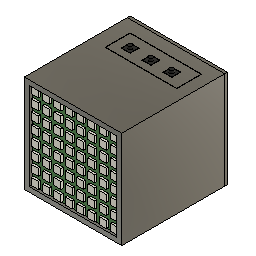
Enclosure (Autodesk Fusion 360 design; units mm, degrees)
Autodesk Fusion 360 part; units mm, degrees
sketch "Sketch1" plane through (0, 0, 0) normal (0, 1, 0) x (1, 0, 0) in component "LED Matrix"
  line L0 (32.5, 32.5) -> (-32.5, 32.5)
  line L1 (-32.5, 32.5) -> (-32.5, -32.5)
  line L2 (-32.5, -32.5) -> (32.5, -32.5)
  line L3 (32.5, -32.5) -> (32.5, 32.5)
  line L4 (32.5, 32.5) -> (-32.5, -32.5) construction
  line L5 (-32.5, 32.5) -> (32.5, -32.5) construction
  line L6 (31, 31) -> (-31, 31)
  line L7 (-31, 31) -> (-31, -31)
  line L8 (-31, -31) -> (31, -31)
  line L9 (31, -31) -> (31, 31)
  dimension "d1" = 65
  dimension "d2" = 65
  constraint parallel L0 L6
  constraint parallel L1 L7
  constraint parallel L2 L8
  constraint parallel L3 L9
  measures "d1" distance of L1.end L2.end
  measures "d2" distance of L0.end L1.end
extrude "Extrude1" add sketch "Sketch1" along normal blind 1.5 contours L0 L1 L2 L3 | L6 L7 L8 L9 makes body 1 in component "LED Matrix"
sketch "Sketch2" plane through (0, 0, 0) normal (0, -1, 0) x (1, 0, 0) in component "LED Matrix"
  line L0 (32.5, -32.5) -> (32.5, 32.5)
  line L1 (32.5, 32.5) -> (-32.5, 32.5)
  line L2 (-32.5, 32.5) -> (-32.5, -32.5)
  line L3 (-32.5, -32.5) -> (32.5, -32.5)
  line L4 (-31, -31) -> (-31, 31)
  line L5 (-31, 31) -> (31, 31)
  line L6 (31, 31) -> (31, -31)
  line L7 (31, -31) -> (-31, -31)
  line L8 (-31, 31) -> (-26, 31)
  line L9 (-26, 31) -> (-26, 26)
  line L10 (-26, 26) -> (-31, 26)
  line L11 (-31, 26) -> (-31, 31)
  line L12 (-22.8571, 31) -> (-17.8571, 31)
  line L13 (-22.8571, 26) -> (-22.8571, 31)
  line L14 (-17.8571, 26) -> (-22.8571, 26)
  line L15 (-17.8571, 31) -> (-17.8571, 26)
  line L16 (-14.7143, 31) -> (-9.7143, 31)
  line L17 (-14.7143, 26) -> (-14.7143, 31)
  line L18 (-9.7143, 26) -> (-14.7143, 26)
  line L19 (-9.7143, 31) -> (-9.7143, 26)
  line L20 (-6.5714, 31) -> (-1.5714, 31)
  line L21 (-6.5714, 26) -> (-6.5714, 31)
  line L22 (-1.5714, 26) -> (-6.5714, 26)
  line L23 (-1.5714, 31) -> (-1.5714, 26)
  line L24 (1.5714, 31) -> (6.5714, 31)
  line L25 (1.5714, 26) -> (1.5714, 31)
  line L26 (6.5714, 26) -> (1.5714, 26)
  line L27 (6.5714, 31) -> (6.5714, 26)
  line L28 (9.7143, 31) -> (14.7143, 31)
  line L29 (9.7143, 26) -> (9.7143, 31)
  line L30 (14.7143, 26) -> (9.7143, 26)
  line L31 (14.7143, 31) -> (14.7143, 26)
  line L32 (17.8571, 31) -> (22.8571, 31)
  line L33 (17.8571, 26) -> (17.8571, 31)
  line L34 (22.8571, 26) -> (17.8571, 26)
  line L35 (22.8571, 31) -> (22.8571, 26)
  line L36 (26, 31) -> (31, 31)
  line L37 (26, 26) -> (26, 31)
  line L38 (31, 26) -> (26, 26)
  line L39 (31, 31) -> (31, 26)
  line L40 (-31, 22.8571) -> (-26, 22.8571)
  line L41 (-31, 17.8571) -> (-31, 22.8571)
  line L42 (-26, 17.8571) -> (-31, 17.8571)
  line L43 (-26, 22.8571) -> (-26, 17.8571)
  line L44 (-22.8571, 22.8571) -> (-17.8571, 22.8571)
  line L45 (-22.8571, 17.8571) -> (-22.8571, 22.8571)
  line L46 (-17.8571, 17.8571) -> (-22.8571, 17.8571)
  line L47 (-17.8571, 22.8571) -> (-17.8571, 17.8571)
  line L48 (-14.7143, 22.8571) -> (-9.7143, 22.8571)
  line L49 (-14.7143, 17.8571) -> (-14.7143, 22.8571)
  line L50 (-9.7143, 17.8571) -> (-14.7143, 17.8571)
  line L51 (-9.7143, 22.8571) -> (-9.7143, 17.8571)
  line L52 (-6.5714, 22.8571) -> (-1.5714, 22.8571)
  line L53 (-6.5714, 17.8571) -> (-6.5714, 22.8571)
  line L54 (-1.5714, 17.8571) -> (-6.5714, 17.8571)
  line L55 (-1.5714, 22.8571) -> (-1.5714, 17.8571)
  line L56 (1.5714, 22.8571) -> (6.5714, 22.8571)
  line L57 (1.5714, 17.8571) -> (1.5714, 22.8571)
  line L58 (6.5714, 17.8571) -> (1.5714, 17.8571)
  line L59 (6.5714, 22.8571) -> (6.5714, 17.8571)
  line L60 (9.7143, 22.8571) -> (14.7143, 22.8571)
  line L61 (9.7143, 17.8571) -> (9.7143, 22.8571)
  line L62 (14.7143, 17.8571) -> (9.7143, 17.8571)
  line L63 (14.7143, 22.8571) -> (14.7143, 17.8571)
  line L64 (17.8571, 22.8571) -> (22.8571, 22.8571)
  line L65 (17.8571, 17.8571) -> (17.8571, 22.8571)
  line L66 (22.8571, 17.8571) -> (17.8571, 17.8571)
  line L67 (22.8571, 22.8571) -> (22.8571, 17.8571)
  line L68 (26, 22.8571) -> (31, 22.8571)
  line L69 (26, 17.8571) -> (26, 22.8571)
  line L70 (31, 17.8571) -> (26, 17.8571)
  line L71 (31, 22.8571) -> (31, 17.8571)
  line L72 (-31, 14.7143) -> (-26, 14.7143)
  line L73 (-31, 9.7143) -> (-31, 14.7143)
  line L74 (-26, 9.7143) -> (-31, 9.7143)
  line L75 (-26, 14.7143) -> (-26, 9.7143)
  line L76 (-22.8571, 14.7143) -> (-17.8571, 14.7143)
  line L77 (-22.8571, 9.7143) -> (-22.8571, 14.7143)
  line L78 (-17.8571, 9.7143) -> (-22.8571, 9.7143)
  line L79 (-17.8571, 14.7143) -> (-17.8571, 9.7143)
  line L80 (-14.7143, 14.7143) -> (-9.7143, 14.7143)
  line L81 (-14.7143, 9.7143) -> (-14.7143, 14.7143)
  line L82 (-9.7143, 9.7143) -> (-14.7143, 9.7143)
  line L83 (-9.7143, 14.7143) -> (-9.7143, 9.7143)
  line L84 (-6.5714, 14.7143) -> (-1.5714, 14.7143)
  line L85 (-6.5714, 9.7143) -> (-6.5714, 14.7143)
  line L86 (-1.5714, 9.7143) -> (-6.5714, 9.7143)
  line L87 (-1.5714, 14.7143) -> (-1.5714, 9.7143)
  line L88 (1.5714, 14.7143) -> (6.5714, 14.7143)
  line L89 (1.5714, 9.7143) -> (1.5714, 14.7143)
  line L90 (6.5714, 9.7143) -> (1.5714, 9.7143)
  line L91 (6.5714, 14.7143) -> (6.5714, 9.7143)
  line L92 (9.7143, 14.7143) -> (14.7143, 14.7143)
  line L93 (9.7143, 9.7143) -> (9.7143, 14.7143)
  line L94 (14.7143, 9.7143) -> (9.7143, 9.7143)
  line L95 (14.7143, 14.7143) -> (14.7143, 9.7143)
  line L96 (17.8571, 14.7143) -> (22.8571, 14.7143)
  line L97 (17.8571, 9.7143) -> (17.8571, 14.7143)
  line L98 (22.8571, 9.7143) -> (17.8571, 9.7143)
  line L99 (22.8571, 14.7143) -> (22.8571, 9.7143)
  line L100 (26, 14.7143) -> (31, 14.7143)
  line L101 (26, 9.7143) -> (26, 14.7143)
  line L102 (31, 9.7143) -> (26, 9.7143)
  line L103 (31, 14.7143) -> (31, 9.7143)
  line L104 (-31, 6.5714) -> (-26, 6.5714)
  line L105 (-31, 1.5714) -> (-31, 6.5714)
  line L106 (-26, 1.5714) -> (-31, 1.5714)
  line L107 (-26, 6.5714) -> (-26, 1.5714)
  line L108 (-22.8571, 6.5714) -> (-17.8571, 6.5714)
  line L109 (-22.8571, 1.5714) -> (-22.8571, 6.5714)
  line L110 (-17.8571, 1.5714) -> (-22.8571, 1.5714)
  line L111 (-17.8571, 6.5714) -> (-17.8571, 1.5714)
  line L112 (-14.7143, 6.5714) -> (-9.7143, 6.5714)
  line L113 (-14.7143, 1.5714) -> (-14.7143, 6.5714)
  line L114 (-9.7143, 1.5714) -> (-14.7143, 1.5714)
  line L115 (-9.7143, 6.5714) -> (-9.7143, 1.5714)
  line L116 (-6.5714, 6.5714) -> (-1.5714, 6.5714)
  line L117 (-6.5714, 1.5714) -> (-6.5714, 6.5714)
  line L118 (-1.5714, 1.5714) -> (-6.5714, 1.5714)
  line L119 (-1.5714, 6.5714) -> (-1.5714, 1.5714)
  line L120 (1.5714, 6.5714) -> (6.5714, 6.5714)
  line L121 (1.5714, 1.5714) -> (1.5714, 6.5714)
  line L122 (6.5714, 1.5714) -> (1.5714, 1.5714)
  line L123 (6.5714, 6.5714) -> (6.5714, 1.5714)
  line L124 (9.7143, 6.5714) -> (14.7143, 6.5714)
  line L125 (9.7143, 1.5714) -> (9.7143, 6.5714)
  line L126 (14.7143, 1.5714) -> (9.7143, 1.5714)
  line L127 (14.7143, 6.5714) -> (14.7143, 1.5714)
  line L128 (17.8571, 6.5714) -> (22.8571, 6.5714)
  line L129 (17.8571, 1.5714) -> (17.8571, 6.5714)
  line L130 (22.8571, 1.5714) -> (17.8571, 1.5714)
  line L131 (22.8571, 6.5714) -> (22.8571, 1.5714)
  line L132 (26, 6.5714) -> (31, 6.5714)
  line L133 (26, 1.5714) -> (26, 6.5714)
  line L134 (31, 1.5714) -> (26, 1.5714)
  line L135 (31, 6.5714) -> (31, 1.5714)
  line L136 (-31, -1.5714) -> (-26, -1.5714)
  line L137 (-31, -6.5714) -> (-31, -1.5714)
  line L138 (-26, -6.5714) -> (-31, -6.5714)
  line L139 (-26, -1.5714) -> (-26, -6.5714)
  line L140 (-22.8571, -1.5714) -> (-17.8571, -1.5714)
  line L141 (-22.8571, -6.5714) -> (-22.8571, -1.5714)
  line L142 (-17.8571, -6.5714) -> (-22.8571, -6.5714)
  line L143 (-17.8571, -1.5714) -> (-17.8571, -6.5714)
  line L144 (-14.7143, -1.5714) -> (-9.7143, -1.5714)
  line L145 (-14.7143, -6.5714) -> (-14.7143, -1.5714)
  line L146 (-9.7143, -6.5714) -> (-14.7143, -6.5714)
  line L147 (-9.7143, -1.5714) -> (-9.7143, -6.5714)
  line L148 (-6.5714, -1.5714) -> (-1.5714, -1.5714)
  line L149 (-6.5714, -6.5714) -> (-6.5714, -1.5714)
  line L150 (-1.5714, -6.5714) -> (-6.5714, -6.5714)
  line L151 (-1.5714, -1.5714) -> (-1.5714, -6.5714)
  line L152 (1.5714, -1.5714) -> (6.5714, -1.5714)
  line L153 (1.5714, -6.5714) -> (1.5714, -1.5714)
  line L154 (6.5714, -6.5714) -> (1.5714, -6.5714)
  line L155 (6.5714, -1.5714) -> (6.5714, -6.5714)
  line L156 (9.7143, -1.5714) -> (14.7143, -1.5714)
  line L157 (9.7143, -6.5714) -> (9.7143, -1.5714)
  line L158 (14.7143, -6.5714) -> (9.7143, -6.5714)
  line L159 (14.7143, -1.5714) -> (14.7143, -6.5714)
  line L160 (17.8571, -1.5714) -> (22.8571, -1.5714)
  line L161 (17.8571, -6.5714) -> (17.8571, -1.5714)
  line L162 (22.8571, -6.5714) -> (17.8571, -6.5714)
  line L163 (22.8571, -1.5714) -> (22.8571, -6.5714)
  line L164 (26, -1.5714) -> (31, -1.5714)
  line L165 (26, -6.5714) -> (26, -1.5714)
  line L166 (31, -6.5714) -> (26, -6.5714)
  line L167 (31, -1.5714) -> (31, -6.5714)
  line L168 (-31, -9.7143) -> (-26, -9.7143)
  line L169 (-31, -14.7143) -> (-31, -9.7143)
  line L170 (-26, -14.7143) -> (-31, -14.7143)
  line L171 (-26, -9.7143) -> (-26, -14.7143)
  line L172 (-22.8571, -9.7143) -> (-17.8571, -9.7143)
  line L173 (-22.8571, -14.7143) -> (-22.8571, -9.7143)
  line L174 (-17.8571, -14.7143) -> (-22.8571, -14.7143)
  line L175 (-17.8571, -9.7143) -> (-17.8571, -14.7143)
  line L176 (-14.7143, -9.7143) -> (-9.7143, -9.7143)
  line L177 (-14.7143, -14.7143) -> (-14.7143, -9.7143)
  line L178 (-9.7143, -14.7143) -> (-14.7143, -14.7143)
  line L179 (-9.7143, -9.7143) -> (-9.7143, -14.7143)
  line L180 (-6.5714, -9.7143) -> (-1.5714, -9.7143)
  line L181 (-6.5714, -14.7143) -> (-6.5714, -9.7143)
  line L182 (-1.5714, -14.7143) -> (-6.5714, -14.7143)
  line L183 (-1.5714, -9.7143) -> (-1.5714, -14.7143)
  line L184 (1.5714, -9.7143) -> (6.5714, -9.7143)
  line L185 (1.5714, -14.7143) -> (1.5714, -9.7143)
  line L186 (6.5714, -14.7143) -> (1.5714, -14.7143)
  line L187 (6.5714, -9.7143) -> (6.5714, -14.7143)
  line L188 (9.7143, -9.7143) -> (14.7143, -9.7143)
  line L189 (9.7143, -14.7143) -> (9.7143, -9.7143)
  line L190 (14.7143, -14.7143) -> (9.7143, -14.7143)
  line L191 (14.7143, -9.7143) -> (14.7143, -14.7143)
  line L192 (17.8571, -9.7143) -> (22.8571, -9.7143)
  line L193 (17.8571, -14.7143) -> (17.8571, -9.7143)
  line L194 (22.8571, -14.7143) -> (17.8571, -14.7143)
  line L195 (22.8571, -9.7143) -> (22.8571, -14.7143)
  line L196 (26, -9.7143) -> (31, -9.7143)
  line L197 (26, -14.7143) -> (26, -9.7143)
  line L198 (31, -14.7143) -> (26, -14.7143)
  line L199 (31, -9.7143) -> (31, -14.7143)
  line L200 (-31, -17.8571) -> (-26, -17.8571)
  line L201 (-31, -22.8571) -> (-31, -17.8571)
  line L202 (-26, -22.8571) -> (-31, -22.8571)
  line L203 (-26, -17.8571) -> (-26, -22.8571)
  line L204 (-22.8571, -17.8571) -> (-17.8571, -17.8571)
  line L205 (-22.8571, -22.8571) -> (-22.8571, -17.8571)
  line L206 (-17.8571, -22.8571) -> (-22.8571, -22.8571)
  line L207 (-17.8571, -17.8571) -> (-17.8571, -22.8571)
  line L208 (-14.7143, -17.8571) -> (-9.7143, -17.8571)
  line L209 (-14.7143, -22.8571) -> (-14.7143, -17.8571)
  line L210 (-9.7143, -22.8571) -> (-14.7143, -22.8571)
  line L211 (-9.7143, -17.8571) -> (-9.7143, -22.8571)
  line L212 (-6.5714, -17.8571) -> (-1.5714, -17.8571)
  line L213 (-6.5714, -22.8571) -> (-6.5714, -17.8571)
  line L214 (-1.5714, -22.8571) -> (-6.5714, -22.8571)
  line L215 (-1.5714, -17.8571) -> (-1.5714, -22.8571)
  line L216 (1.5714, -17.8571) -> (6.5714, -17.8571)
  line L217 (1.5714, -22.8571) -> (1.5714, -17.8571)
  line L218 (6.5714, -22.8571) -> (1.5714, -22.8571)
  line L219 (6.5714, -17.8571) -> (6.5714, -22.8571)
  line L220 (9.7143, -17.8571) -> (14.7143, -17.8571)
  line L221 (9.7143, -22.8571) -> (9.7143, -17.8571)
  line L222 (14.7143, -22.8571) -> (9.7143, -22.8571)
  line L223 (14.7143, -17.8571) -> (14.7143, -22.8571)
  line L224 (17.8571, -17.8571) -> (22.8571, -17.8571)
  line L225 (17.8571, -22.8571) -> (17.8571, -17.8571)
  line L226 (22.8571, -22.8571) -> (17.8571, -22.8571)
  line L227 (22.8571, -17.8571) -> (22.8571, -22.8571)
  line L228 (26, -17.8571) -> (31, -17.8571)
  line L229 (26, -22.8571) -> (26, -17.8571)
  line L230 (31, -22.8571) -> (26, -22.8571)
  line L231 (31, -17.8571) -> (31, -22.8571)
  line L232 (-31, -26) -> (-26, -26)
  line L233 (-31, -31) -> (-31, -26)
  line L234 (-26, -31) -> (-31, -31)
  line L235 (-26, -26) -> (-26, -31)
  line L236 (-22.8571, -26) -> (-17.8571, -26)
  line L237 (-22.8571, -31) -> (-22.8571, -26)
  line L238 (-17.8571, -31) -> (-22.8571, -31)
  line L239 (-17.8571, -26) -> (-17.8571, -31)
  line L240 (-14.7143, -26) -> (-9.7143, -26)
  line L241 (-14.7143, -31) -> (-14.7143, -26)
  line L242 (-9.7143, -31) -> (-14.7143, -31)
  line L243 (-9.7143, -26) -> (-9.7143, -31)
  line L244 (-6.5714, -26) -> (-1.5714, -26)
  line L245 (-6.5714, -31) -> (-6.5714, -26)
  line L246 (-1.5714, -31) -> (-6.5714, -31)
  line L247 (-1.5714, -26) -> (-1.5714, -31)
  line L248 (1.5714, -26) -> (6.5714, -26)
  line L249 (1.5714, -31) -> (1.5714, -26)
  line L250 (6.5714, -31) -> (1.5714, -31)
  line L251 (6.5714, -26) -> (6.5714, -31)
  line L252 (9.7143, -26) -> (14.7143, -26)
  line L253 (9.7143, -31) -> (9.7143, -26)
  line L254 (14.7143, -31) -> (9.7143, -31)
  line L255 (14.7143, -26) -> (14.7143, -31)
  line L256 (17.8571, -26) -> (22.8571, -26)
  line L257 (17.8571, -31) -> (17.8571, -26)
  line L258 (22.8571, -31) -> (17.8571, -31)
  line L259 (22.8571, -26) -> (22.8571, -31)
  line L260 (26, -26) -> (31, -26)
  line L261 (26, -31) -> (26, -26)
  line L262 (31, -31) -> (26, -31)
  line L263 (31, -26) -> (31, -31)
  dimension "d12" = 57
  dimension "d13" = -57
  constraint horizontal L8
  constraint vertical L9
  constraint horizontal L10
  constraint vertical L11
  constraint coincident L4.end L5.start
extrude "Extrude2" add sketch "Sketch2" along normal blind 1.5 separate body contours L4 L7 L232 L233 L234 L235 | L4 L200 L201 L202 L203 | L7 L236 L237 L238 L239 | L4 L168 L169 L170 L171 | L7 L240 L241 L242 L243 | L4 L136 L137 L138 L139 | L7 L244 L245 L246 L247 | L4 L104 L105 L106 L107 | L7 L248 L249 L250 L251 | L4 L72 L73 L74 L75 | L7 L252 L253 L254 L255 | L4 L40 L41 L42 L43 | L7 L256 L257 L258 L259 | L4 L5 L8 L9 L10 L11 | L6 L7 L260 L261 L262 L263 | L5 L12 L13 L14 L15 | L6 L228 L229 L230 L231 | L5 L16 L17 L18 L19 | L6 L196 L197 L198 L199 | L5 L20 L21 L22 L23 | L6 L164 L165 L166 L167 | L5 L24 L25 L26 L27 | L6 L132 L133 L134 L135 | L5 L28 L29 L30 L31 | L6 L100 L101 L102 L103 | L5 L32 L33 L34 L35 | L6 L68 L69 L70 L71 | L5 L6 L36 L37 L38 L39 | L44 L45 L46 L47 | L48 L49 L50 L51 | L52 L53 L54 L55 | L56 L57 L58 L59 | L60 L61 L62 L63 | L64 L65 L66 L67 | L76 L77 L78 L79 | L80 L81 L82 L83 | L84 L85 L86 L87 | L88 L89 L90 L91 | L92 L93 L94 L95 | L96 L97 L98 L99 | L108 L109 L110 L111 | L112 L113 L114 L115 | L116 L117 L118 L119 | L120 L121 L122 L123 | L124 L125 L126 L127 | L128 L129 L130 L131 | L140 L141 L142 L143 | L144 L145 L146 L147 | L148 L149 L150 L151 | L152 L153 L154 L155 | L156 L157 L158 L159 | L160 L161 L162 L163 | L172 L173 L174 L175 | L176 L177 L178 L179 | L180 L181 L182 L183 | L184 L185 L186 L187 | L188 L189 L190 L191 | L192 L193 L194 L195 | L204 L205 L206 L207 | L208 L209 L210 L211 | L212 L213 L214 L215 | L216 L217 L218 L219 | L220 L221 L222 L223 | L224 L225 L226 L227 makes body 2 at (11.381, 0, -27.6667) makes body 3 at (-19.5238, 0, -27.6667) makes body 4 at (-13.0476, 0, -19.5238) makes body 5 at (19.5238, 0, -19.5238) makes body 6 at (11.381, 0, -11.381) makes body 7 at (-19.5238, 0, -11.381) makes body 8 at (-13.0476, 0, -3.2381) makes body 9 at (19.5238, 0, -3.2381) makes body 10 at (11.381, 0, 4.9048) makes body 11 at (-19.5238, 0, 4.9048) makes body 12 at (11.381, 0, 13.0476) makes body 13 at (-19.5238, 0, 13.0476) makes body 14 at (-13.0476, 0, 21.1905) makes body 15 at (19.5238, 0, 21.1905) makes body 16 at (11.381, 0, 29.3333) makes body 17 at (-19.5238, 0, 29.3333) makes body 18 at (-13.0476, 0, 29.3333) makes body 19 at (19.5238, 0, 29.3333) makes body 20 at (11.381, 0, 21.1905) makes body 21 at (-19.5238, 0, 21.1905) makes body 22 at (-13.0476, 0, 13.0476) makes body 23 at (19.5238, 0, 13.0476) makes body 24 at (-13.0476, 0, 4.9048) makes body 25 at (19.5238, 0, 4.9048) makes body 26 at (11.381, 0, -3.2381) makes body 27 at (-19.5238, 0, -3.2381) makes body 28 at (-13.0476, 0, -11.381) makes body 29 at (19.5238, 0, -11.381) makes body 30 at (11.381, 0, -19.5238) makes body 31 at (-19.5238, 0, -19.5238) makes body 32 at (-13.0476, 0, -27.6667) makes body 33 at (19.5238, 0, -27.6667) makes body 34 at (3.2381, 0, -29.3333) makes body 35 at (-29.3333, 0, -27.6667) makes body 36 at (-4.9048, 0, -19.5238) makes body 37 at (27.6667, 0, -19.5238) makes body 38 at (3.2381, 0, -11.381) makes body 39 at (-29.3333, 0, -11.381) makes body 40 at (-4.9048, 0, -3.2381) makes body 41 at (27.6667, 0, -4.9048) makes body 42 at (3.2381, 0, 4.9048) makes body 43 at (-29.3333, 0, 4.9048) makes body 44 at (4.9048, 0, 11.381) makes body 45 at (-29.3333, 0, 13.0476) makes body 46 at (-4.9048, 0, 21.1905) makes body 47 at (27.6667, 0, 21.1905) makes body 48 at (3.2381, 0, 29.3333) makes body 49 at (-29.3333, 0, 29.3333) makes body 50 at (-4.9048, 0, 29.3333) makes body 51 at (29.3333, 0, 29.3333) makes body 52 at (3.2381, 0, 21.1905) makes body 53 at (-29.3333, 0, 21.1905) makes body 54 at (-3.2381, 0, 11.381) makes body 55 at (27.6667, 0, 11.381) makes body 56 at (-4.9048, 0, 4.9048) makes body 57 at (27.6667, 0, 4.9048) makes body 58 at (3.2381, 0, -3.2381) makes body 59 at (-29.3333, 0, -3.2381) makes body 60 at (-4.9048, 0, -11.381) makes body 61 at (29.3333, 0, -13.0476) makes body 62 at (3.2381, 0, -19.5238) makes body 63 at (-29.3333, 0, -19.5238) makes body 64 at (-4.9048, 0, -27.6667) makes body 65 at (29.3333, 0, -29.3333) in component "LED Matrix"
sketch "Sketch3" plane through (0, 1.5, 0) normal (0, 1, 0) x (-1, 0, 0) in component "LED Matrix"
  line L0 (-32.5, 32.5) -> (-32.5, -32.5)
  line L1 (-32.5, -32.5) -> (32.5, -32.5)
  line L2 (32.5, -32.5) -> (32.5, 32.5)
  line L3 (32.5, 32.5) -> (-32.5, 32.5)
  line L4 (24.5, -32.5) -> (24.5, 32.5) construction
  line L5 (32.5, 25.8) -> (-32.5, 25.8) construction
  line L6 (24.5, 25.8) -> (32.5, 25.8)
  line L7 (32.5, 25.8) -> (32.5, 23.3)
  line L8 (32.5, 23.3) -> (24.5, 23.3)
  line L9 (24.5, 23.3) -> (24.5, 25.8)
  dimension "d117" = -8
  dimension "d118" = -6.7
  dimension "d119" = 2.5
  constraint horizontal L6
  constraint vertical L7
  constraint horizontal L8
  constraint vertical L9
  constraint coincident L4 L6.start
  constraint coincident L5 L6.start
  measures "d119" distance of L6.start L8.end
extrude "Extrude3" add sketch "Sketch3" along normal blind 18 separate body contours L2 L6 L7 L8 L9 makes body 66 in component "LED Matrix"
sketch "Sketch1 (2)" plane through (0, 1.5, 0) normal (0, 1, 0) x (-1, 0, 0) in component "Box"
  line L0 (-32.5, 32.5) -> (-32.5, -32.5)
  line L1 (-32.5, -32.5) -> (32.5, -32.5)
  line L2 (32.5, -32.5) -> (32.5, 32.5)
  line L3 (32.5, 32.5) -> (-32.5, 32.5)
  line L4 (-33, -33) -> (33, -33)
  line L5 (33, -33) -> (33, 33)
  line L6 (33, 33) -> (-33, 33)
  line L7 (-33, 33) -> (-33, -33)
  line L8 (-35, -35) -> (35, -35)
  line L9 (35, -35) -> (35, 35)
  line L10 (35, 35) -> (-35, 35)
  line L11 (-35, 35) -> (-35, -35)
  line L12 (-26, 31) -> (-31, 31)
  line L13 (-31, 31) -> (-31, 26)
  line L14 (-31, 26) -> (-26, 26)
  line L15 (-26, 26) -> (-26, 31)
  line L16 (31, -26) -> (26, -26)
  line L17 (26, -26) -> (26, -31)
  line L18 (26, -31) -> (31, -31)
  line L19 (31, -31) -> (31, -26)
  line L20 (-31, 31) -> (31, 31) construction
  line L21 (31, 31) -> (31, -31) construction
  line L22 (31, -31) -> (-31, -31) construction
  line L23 (-31, -31) -> (-31, 31) construction
  line L24 (31.5, -31.5) -> (-31.5, -31.5)
  line L25 (-31.5, -31.5) -> (-31.5, 31.5)
  line L26 (-31.5, 31.5) -> (31.5, 31.5)
  line L27 (31.5, 31.5) -> (31.5, -31.5)
  dimension "d16" = 0.5
  dimension "d17" = 2.5
  dimension "d18" = -0.5
  constraint horizontal L20
  constraint vertical L21
  constraint horizontal L22
  constraint vertical L23
  constraint coincident L18.end L19.start
  constraint coincident L12.end L13.start
extrude "Extrude1'" add sketch "Sketch1 (2)" against normal blind 4 separate body contours L8 L9 L10 L11 makes body 67 in component "Box"
extrude "Extrude2'" add sketch "Sketch1 (2)" against normal up to surface (2 mm away) from surface at -2 contours L0 L1 L2 L3 | L4 L5 L6 L7 bodies 67 in component "Box"
extrude "Extrude3'" add 1 faces at (-11, 1.5, -34.3333) along direction (0, 1, 0) blind 2 on bodies 67 bodies 67 in component "Box"
sketch "Sketch2 (2)" plane through (0, 3.5, 0) normal (0, 1, 0) x (-1, 0, 0) in component "Box"
  line L0 (-33, -33) -> (-33, 33)
  line L1 (-33, 33) -> (33, 33)
  line L2 (33, 33) -> (33, -33)
  line L3 (33, -33) -> (-33, -33)
  line L4 (-35, 35) -> (-35, -35)
  line L5 (-35, -35) -> (35, -35)
  line L6 (35, -35) -> (35, 35)
  line L7 (35, 35) -> (-35, 35)
  line L8 (35, -35) -> (-35, -35)
  line L9 (-35, -35) -> (-35, 35)
  line L10 (-35, 35) -> (35, 35)
  line L11 (35, 35) -> (35, -35)
  dimension "d30" = -2
extrude "Extrude4" add sketch "Sketch2 (2)" along normal blind 68 bodies 67 in component "Box"
sketch "Sketch1 (3)" plane through (0, 0, -33) normal (0, 0, 1) x (-1, 0, 0) in component "Arduino"
  line L0 (34.6, -34.5) -> (-29.4, -34.5) construction
  line L1 (-26.6, -35) -> (-26.6, 35) construction
  line L2 (-26.6, -34.5) -> (-26.6, 34.5)
  line L3 (-26.6, 34.5) -> (26.6, 34.5)
  line L4 (26.6, 34.5) -> (26.6, -34.5)
  line L5 (26.6, -34.5) -> (-26.6, -34.5)
  line L6 (-18.1, -35) -> (-18.1, 35) construction
  line L7 (-5.1, -35) -> (-5.1, 34.5) construction
  line L8 (23.1, 34.5) -> (23.1, -34.5) construction
  line L9 (13.1, -34.5) -> (13.1, 34.5) construction
  line L10 (25.8, -34.5) -> (25.8, 34.5) construction
  line L11 (26.6, -22.2) -> (-26.6, -22.2) construction
  line L12 (20.8, -34.5) -> (20.8, 34.5) construction
  circle A0 centre (24.3, -20.7) radius 1.5
  line L13 (-25.8, -34.5) -> (-25.8, 34.5) construction
  line L14 (-26.6, -21) -> (26.6, -21) construction
  circle A1 centre (-24.3, -19.5) radius 1.5
  line L15 (-10.1, -34.5) -> (-10.1, 34.5) construction
  line L16 (-26.6, 33.7) -> (26.6, 33.7) construction
  circle A2 centre (19.3, 32.2) radius 1.5
  circle A3 centre (-8.6, 32.2) radius 1.5
  line L17 (-7.1, -34.5) -> (-7.1, 34.5) construction
  line L18 (17.8, -34.5) -> (17.8, 34.5) construction
  line L19 (-18.1, -35) -> (-5.1, -35) construction
  line L20 (-5.6, -40) -> (-5.6, -23.8)
  line L21 (-5.6, -23.8) -> (-17.6, -23.8)
  line L22 (-17.6, -23.8) -> (-17.6, -40)
  line L23 (-5.6, -40) -> (-17.6, -40)
  line L24 (23.1, -34.5) -> (13.1, -34.5)
  line L25 (13.6, -36.3) -> (13.6, -22.3)
  line L26 (13.6, -22.3) -> (22.6, -22.3)
  line L27 (22.6, -22.3) -> (22.6, -36.3)
  line L28 (13.6, -36.3) -> (22.6, -36.3)
  line L29 (26.6, 34.5) -> (-26.6, -34.5) construction
  line L30 (26.6, -34.5) -> (-26.6, 34.5) construction
  dimension "d35" = 69
  dimension "d36" = 53.2
  dimension "d38" = 13
  dimension "d40" = 10
  dimension "d41" = 12.3
  dimension "d42" = 0.8
  dimension "d44" = 0.8
  dimension "d45" = 13.5
  dimension "d49" = 3
  dimension "d50" = 3
  dimension "d51" = 5.8
  dimension "d52" = 0.8
  dimension "d54" = 3
  dimension "d55" = 16.5
  dimension "d57" = 3
  dimension "d60" = 24.9
  dimension "d64" = 10.7
  dimension "d65" = 0.5
  dimension "d66" = 0.5
  dimension "d72" = 0.5
  dimension "d73" = 0.5
  dimension "d74" = 12.2
  constraint coincident L0 L2.start
  constraint coincident L1 L2.start
  constraint coincident L3 L7.end
  constraint perpendicular L3 L7
  constraint coincident L0 L9.start
  constraint coincident L3 L9.end
  constraint perpendicular L3 L9
  constraint coincident L0 L10.start
  constraint coincident L3 L10.end
  constraint perpendicular L3 L10
  constraint coincident L4 L11.start
  constraint coincident L1 L11.end
  constraint coincident L0 L12.start
  constraint coincident L3 L12.end
  constraint perpendicular L3 L12
  constraint tangent L11 A0
  constraint tangent L10 A0
  constraint coincident L5 L13.start
  constraint coincident L3 L13.end
  constraint perpendicular L3 L13
  constraint coincident L1 L14.start
  constraint coincident L4 L14.end
  constraint perpendicular L4 L14
  constraint tangent L13 A1
  constraint tangent L14 A1
  constraint coincident L0 L15.start
  constraint coincident L3 L15.end
  constraint perpendicular L3 L15
  constraint coincident L1 L16.start
  constraint coincident L4 L16.end
  constraint perpendicular L4 L16
  constraint tangent L16 A2
  constraint tangent L12 A2
  constraint tangent L15 A3
  constraint tangent L16 A3
  constraint midpoint L29 origin
  constraint parallel L1 L6
  constraint parallel L4 L8
  constraint parallel L12 L18
  constraint parallel L15 L17
  constraint parallel L21 L23
  constraint parallel L26 L28
  measures "d35" distance of L2.start L2.end
  measures "d36" distance of L2.start L4.end
  measures "d38" distance of L6 L7
  measures "d40" distance of L8 L9
  measures "d41" distance of L5 L11
  measures "d42" distance of L4 L10
  measures "d44" distance of L1 L13
  measures "d45" distance of L0 L14
  measures "d49" diameter of A1
  measures "d50" diameter of A0
  measures "d51" distance of L4 L12
  measures "d52" distance of L3 L16
  measures "d54" diameter of A2
  measures "d55" distance of L2 L15
  measures "d57" diameter of A3
  measures "d60" distance of L17 L18
  measures "d64" distance of L5 L21
  measures "d65" distance of L7 L20
  measures "d66" distance of L6 L22
  measures "d72" distance of L8 L27
  measures "d73" distance of L9 L25
  measures "d74" distance of L24 L26
extrude "Extrude1''" add sketch "Sketch1 (3)" along normal blind 1.5 separate body contours L2 L3 L4 L5 L20 L21 L22 L24 L25 L26 L27 | L5 L20 L21 L22 | L5 L24 L25 L26 L27 makes body 68 in component "Arduino"
extrude "Extrude2''" add sketch "Sketch1 (3)" along normal blind 11 from surface at 1.5 separate body contours L5 L20 L21 L22 | L5 L20 L22 L23 makes body 69 in component "Arduino"
extrude "Extrude3''" add sketch "Sketch1 (3)" along normal blind 11 from surface at 1.5 separate body contours L5 L24 L25 L26 L27 | L5 L24 L25 L27 L28 makes body 70 in component "Arduino"
sketch "Sketch2 (3)" plane through (0, 0, -31.5) normal (0, 0, 1) x (-1, 0, 0) in component "Arduino"
  circle A0 centre (24.3, -20.7) radius 1.5
  circle A1 centre (19.3, 32.2) radius 1.5
  circle A2 centre (-24.3, -19.5) radius 1.5
  circle A3 centre (-8.6, 32.2) radius 1.5
  line L0 (26.6, -34.5) -> (26.6, 34.5)
  line L1 (26.6, 34.5) -> (-26.6, 34.5)
  line L2 (-26.6, 34.5) -> (-26.6, -34.5)
  line L3 (-26.6, -34.5) -> (26.6, -34.5)
  line L4 (-26.6, -17.5) -> (26.6, -17.5) construction
  line L5 (-26.6, -13) -> (26.6, -13) construction
  line L6 (25.8, -34.5) -> (25.8, 34.5)
  line L7 (-25.8, -34.5) -> (-25.8, 34.5)
  line L8 (-26.6, -13) -> (26.6, -13) construction
  line L9 (-26.6, -17.5) -> (26.6, -17.5) construction
  line L10 (24.3, -20.7) -> (24.3, 34.5) construction
  line L11 (-24.3, -19.5) -> (-24.3, 34.5) construction
  line L12 (26.6, 30.5) -> (-26.6, 30.5) construction
  line L13 (25.8, -13) -> (22.8, -13)
  line L14 (22.8, -13) -> (22.8, 30.5)
  line L15 (22.8, 30.5) -> (25.8, 30.5)
  line L16 (25.8, 30.5) -> (25.8, -13)
  line L17 (-25.8, -17.5) -> (-22.8, -17.5)
  line L18 (-22.8, -17.5) -> (-22.8, 30.5)
  line L19 (-22.8, 30.5) -> (-25.8, 30.5)
  line L20 (-25.8, 30.5) -> (-25.8, -17.5)
  circle A4 centre (24.3, -20.7) radius 1.5
  circle A5 centre (-24.3, -19.5) radius 1.5
  circle A6 centre (-8.6, 32.2) radius 1.5
  circle A7 centre (19.3, 32.2) radius 1.5
  line L21 (26.6, -34.5) -> (26.6, 34.5)
  line L22 (26.6, 34.5) -> (-26.6, 34.5)
  line L23 (-26.6, 34.5) -> (-26.6, -34.5)
  line L24 (-26.6, -34.5) -> (26.6, -34.5)
  dimension "d164" = -21.5
  dimension "d165" = -17
  dimension "d167" = 48
  dimension "d168" = 3
  dimension "d169" = 3
  constraint coincident A0.centre L10.start
  constraint coincident L1 L10.end
  constraint perpendicular L1 L10
  constraint coincident A2.centre L11.start
  constraint coincident L1 L11.end
  constraint perpendicular L1 L11
  constraint coincident L0 L12.start
  constraint coincident L2 L12.end
  constraint perpendicular L2 L12
  constraint horizontal L13
  constraint vertical L14
  constraint horizontal L15
  constraint vertical L16
  constraint coincident L5 L13.start
  constraint coincident L6 L13.start
  constraint collinear L12 L15
  constraint horizontal L17
  constraint vertical L18
  constraint horizontal L19
  constraint vertical L20
  constraint coincident L4 L17.start
  constraint coincident L7 L17.start
  constraint collinear L12 L19
  measures "d167" distance of L9 L12
  measures "d168" distance of L13.start L13.end
  measures "d169" distance of L17.start L17.end
extrude "Extrude4'" add sketch "Sketch2 (3)" along normal blind 8.5 separate body contours L6 L13 L14 L15 L16 | L7 L17 L18 L19 L20 makes body 71 at (-22.8, -1.5, -28.6667) makes body 72 at (25.8, 1.5, -28.6667) in component "Arduino"
sketch "Sketch4" plane through (0, 36.5, -33) normal (0, 0, 1) x (-1, 0, 0) in component "Box"
  circle A0 centre (-24.3, -19.5) radius 2.5
  circle A1 centre (24.3, -20.7) radius 2.5
  circle A2 centre (24.3, -20.7) radius 1.5
  circle A3 centre (-24.3, -19.5) radius 1.5
  circle A4 centre (19.3, 32.2) radius 1.5
  circle A5 centre (-8.6, 32.2) radius 1.5
  line L0 (19.3, 32.2) -> (-8.6, 32.2) construction
  line L1 (21.5913, 33.2) -> (-10.8913, 33.2)
  arc A6 (17.0087, 33.2) -> (21.5913, 33.2) centre (19.3, 32.2) ccw
  arc A7 (-10.8913, 33.2) -> (-6.3087, 33.2) centre (-8.6, 32.2) ccw
  circle A8 centre (24.3, -20.7) radius 1
  circle A9 centre (-24.3, -19.5) radius 1
  circle A10 centre (19.3, 32.2) radius 1
  circle A11 centre (-8.6, 32.2) radius 1
  dimension "d170" = 1
  dimension "d171" = 1
  dimension "d172" = 1
  dimension "d173" = 1
  dimension "d249" = -0.5
  dimension "d250" = -0.5
  dimension "d251" = -0.5
  dimension "d252" = -0.5
  constraint coincident A4.centre L0.start
  constraint coincident A5.centre L0.end
  constraint parallel L0 L1
  constraint coincident L1 A6.start
  constraint coincident L1 A7.end
  constraint tangent L1 A10
  measures "d170" distance of A1 A2
  measures "d171" distance of A0 A3
  measures "d172" distance of A4 A6
  measures "d173" distance of A5 A7
extrude "Extrude5" add sketch "Sketch4" along normal up to surface (5 mm away) contours A0 | A1 | A2 | A3 | A10 | A4 L1 | A4 L1 A6 | A11 | A5 L1 | A5 L1 A7 | A8 | A9 picked at (18.2516, 33.0192) picked at (-9.6484, 33.0192) bodies 67 in component "Box"
extrude "Extrude6" add sketch "Sketch4" along normal blind 7 contours A10 | A11 | A8 | A9 bodies 67 in component "Box"
sketch "Sketch1 (4)" plane through (0, 71.5, 0) normal (0, 1, 0) x (-1, 0, 0) in component "Door"
  line L0 (35, 35) -> (-35, 35)
  line L1 (-35, 35) -> (-35, -35)
  line L2 (-35, -35) -> (35, -35)
  line L3 (35, -35) -> (35, 35)
  line L4 (34.5, -34.5) -> (-34.5, -34.5)
  line L5 (-34.5, -34.5) -> (-34.5, 34.5)
  line L6 (-34.5, 34.5) -> (34.5, 34.5)
  line L7 (34.5, 34.5) -> (34.5, -34.5)
  line L8 (33, 33) -> (33, -33)
  line L9 (33, -33) -> (-33, -33)
  line L10 (-33, -33) -> (-33, 33)
  line L11 (-33, 33) -> (33, 33)
extrude "Extrude1'''" add sketch "Sketch1 (4)" along normal blind 2 separate body contours L0 L1 L2 L3 | L4 L5 L6 L7 | L8 L9 L10 L11 makes body 73 in component "Door"
extrude "Extrude2'''" add sketch "Sketch1 (4)" against normal blind 2 contours L8 L9 L10 L11 bodies 73 in component "Door"
draft "Draft1" angle 11.25 neutral plane through (0, 71.5, 0) pull (0, -1, 0) 4 faces at (11, 70.1667, 33) (33, 70.1667, -11) (-11, 70.1667, -33) (-33, 70.1667, 11) on bodies 73 in component "Door"
sketch "Sketch4 (2)" plane through (0, 73.5, 0) normal (0, 1, 0) x (-1, 0, 0) in component "Door"
  line L0 (35, -35) -> (35, 35)
  line L1 (35, 35) -> (-35, 35)
  line L2 (-35, 35) -> (-35, -35)
  line L3 (-35, -35) -> (35, -35)
  line L4 (-17.6, -26.5) -> (-5.6, -26.5)
  line L5 (-5.6, -26.5) -> (-5.6, -15.5)
  line L6 (-5.6, -15.5) -> (-17.6, -15.5)
  line L7 (-17.6, -15.5) -> (-17.6, -26.5)
  line L8 (13.6, -26.5) -> (22.6, -26.5)
  line L9 (22.6, -26.5) -> (22.6, -15.5)
  line L10 (22.6, -15.5) -> (13.6, -15.5)
  line L11 (13.6, -15.5) -> (13.6, -26.5)
  line L12 (-18.1, -27) -> (-5.1, -27)
  line L13 (-5.1, -27) -> (-5.1, -15)
  line L14 (-5.1, -15) -> (-18.1, -15)
  line L15 (-18.1, -15) -> (-18.1, -27)
  line L16 (13.1, -27) -> (23.1, -27)
  line L17 (23.1, -27) -> (23.1, -15)
  line L18 (23.1, -15) -> (13.1, -15)
  line L19 (13.1, -15) -> (13.1, -27)
  dimension "d174" = 0.5
  dimension "d175" = 0.5
extrude "Extrude4''" cut sketch "Sketch4 (2)" against normal up to surface (4 mm away) contours L4 L5 L6 L7 | L8 L9 L10 L11 | L12 L13 L14 L15 | L16 L17 L18 L19 bodies 73 in component "Door"
draft "Draft2" angle -11.25 neutral plane through (0, 73.5, 0) pull (0, 1, 0) 8 faces at (9.4333, 72.1667, -15) (5.1, 72.1667, -23) (-19.7667, 70.8333, -15) (-23.1, 72.1667, -23) (18.1, 72.1667, -19) (13.7667, 70.8333, -27) (-13.1, 72.1667, -19) (-16.4333, 72.1667, -27) on bodies 73 in component "Door"
sketch "Sketch3 (2)" plane through (0, 73.5, 0) normal (0, 1, 0) x (-1, 0, 0) in component "Door"
  line L0 (35, -35) -> (35, 35)
  line L1 (35, 35) -> (-35, 35)
  line L2 (-35, 35) -> (-35, -35)
  line L3 (-35, -35) -> (35, -35)
  line L4 (0, 34.1022) -> (0, -34.1022) construction
  line L5 (-23, -23) -> (23, -23) construction
  line L6 (23, -23) -> (23, 23) construction
  line L7 (23, 23) -> (-23, 23) construction
  line L8 (-23, 23) -> (-23, -23) construction
  line L9 (-4, 34.1022) -> (-4, -34.1022) construction
  line L10 (4, 34.1022) -> (4, -34.1022) construction
  line L11 (-21, 21) -> (-6, 21)
  arc A0 (-6, 21) -> (-6, 25) centre (-6, 23) ccw
  line L12 (-6, 25) -> (-21, 25)
  arc A1 (-21, 25) -> (-21, 21) centre (-21, 23) ccw
  line L13 (-23, 23) -> (-4, 23) construction
  line L14 (22, 25) -> (7, 25)
  arc A2 (7, 25) -> (7, 21) centre (7, 23) ccw
  line L15 (7, 21) -> (22, 21)
  arc A3 (22, 21) -> (22, 25) centre (22, 23) ccw
  line L16 (-18.1, -15) -> (-5.1, -15)
  line L17 (-5.1, -15) -> (-5.1, -27)
  line L18 (-5.1, -27) -> (-18.1, -27)
  line L19 (-18.1, -27) -> (-18.1, -15)
  line L20 (13.1, -15) -> (23.1, -15)
  line L21 (23.1, -15) -> (23.1, -27)
  line L22 (23.1, -27) -> (13.1, -27)
  line L23 (13.1, -27) -> (13.1, -15)
  line L24 (-4.3044, -14.2044) -> (-18.8956, -14.2044)
  line L25 (-18.8956, -14.2044) -> (-18.8956, -27.7956)
  line L26 (-18.8956, -27.7956) -> (-4.3044, -27.7956)
  line L27 (-4.3044, -27.7956) -> (-4.3044, -14.2044)
  line L28 (23.8956, -14.2044) -> (12.3044, -14.2044)
  line L29 (12.3044, -14.2044) -> (12.3044, -27.7956)
  line L30 (12.3044, -27.7956) -> (23.8956, -27.7956)
  line L31 (23.8956, -27.7956) -> (23.8956, -14.2044)
  line L32 (-32.6022, -32.6022) -> (-32.6022, 32.6022)
  line L33 (-32.6022, 32.6022) -> (32.6022, 32.6022)
  line L34 (32.6022, 32.6022) -> (32.6022, -32.6022)
  line L35 (32.6022, -32.6022) -> (-32.6022, -32.6022)
  dimension "d107" = -12
  dimension "d108" = 4
  dimension "d109" = -4
  dimension "d112" = 28
  dimension "d113" = -48
  dimension "d114" = 4
  dimension "d180" = 70
  dimension "d181" = 70
  constraint tangent L11 A0
  constraint tangent A0 L12
  constraint parallel L11 L12
  constraint tangent L12 A1
  constraint tangent L11 A1
  constraint midpoint L7.end A1
  constraint midpoint A0 L13.end
  constraint coincident L9 L13.end
  constraint coincident L7 L13.end
  measures "d114" distance of L11 L12
  measures "d180" distance of L1.end L2.end
  measures "d181" distance of L0.end L1.end
extrude "Extrude3'''" cut sketch "Sketch3 (2)" against normal up to surface (4 mm away) contours L11 A0 L12 A1 | L14 A2 L15 A3 bodies 73 in component "Door"
sketch "Sketch1 (5)" plane through (0, 0, 0) normal (0, 0, 1) x (1, 0, 0) in component "Buttons"
  line L0 (-23, 8) -> (-23, -7)
  line L1 (25.5, -7) -> (25.5, 8)
  line L2 (-23, 8) -> (25.5, 8)
  line L3 (-23, -7) -> (25.5, -7)
  line L4 (3, 3) -> (-3, 3)
  line L5 (-3, 3) -> (-3, -3)
  line L6 (-3, -3) -> (3, -3)
  line L7 (3, -3) -> (3, 3)
  line L8 (3, 3) -> (-3, -3) construction
  line L9 (-3, 3) -> (3, -3) construction
  circle A0 centre (0, 0) radius 1.5
  line L10 (-18, -3) -> (-12, -3)
  line L11 (-12, 3) -> (-18, 3)
  line L12 (-18, 3) -> (-12, -3) construction
  line L13 (-12, 3) -> (-18, -3) construction
  circle A1 centre (-15, 0) radius 1.5
  line L14 (-18, 3) -> (-18, -3)
  line L15 (-12, -3) -> (-12, 3)
  line L16 (12, -3) -> (18, -3)
  line L17 (18, 3) -> (12, 3)
  line L18 (12, 3) -> (18, -3) construction
  line L19 (18, 3) -> (12, -3) construction
  circle A2 centre (15, 0) radius 1.5
  line L20 (12, 3) -> (12, -3)
  line L21 (18, -3) -> (18, 3)
  line L22 (-23, 8) -> (-20, 8)
  line L23 (-20, 8) -> (-20, -3)
  line L24 (-20, -3) -> (-23, -3)
  line L25 (-23, -3) -> (-23, 8)
  point P0 (-15, 0)
  point P1 (-15, 0)
  point P2 (15, 0)
  point P3 (15, 0)
  dimension "d154" = 15
  dimension "d187" = 6
  dimension "d188" = 6
  dimension "d189" = 3
  dimension "d192" = 15
  dimension "d193" = 0
  dimension "d194" = 5
  dimension "d195" = 7.5
  dimension "d196" = 5
  dimension "d203" = 3
  dimension "d204" = 11
  constraint horizontal L4
  constraint perpendicular L4 L5
  constraint parallel L4 L6
  constraint parallel L5 L7
  constraint coincident L8 A0.centre
  constraint coincident L9 A0.centre
  constraint coincident A0.centre origin
  constraint horizontal L22
  constraint vertical L23
  constraint horizontal L24
  constraint vertical L25
  measures "d187" distance of L5.end L6.end
  measures "d188" distance of L4.end L5.end
  measures "d189" diameter of A0
  measures "d194" distance of L0 L14
  measures "d195" distance of L1 L21
  measures "d196" distance of L2 L4
  measures "d203" distance of L0.start L22.end
  measures "d204" distance of L0.start L24.end
extrude "Extrude2''''" add sketch "Sketch1 (5)" along normal blind 1.5 separate body contours L0 L2 L22 L23 L24 L25 | L0 L1 L2 L3 L23 L24 | L4 L5 L6 L7 | A0 | L10 L11 L14 L15 | A1 | L16 L17 L20 L21 | A2 makes body 74 in component "Buttons"
extrude "Extrude1''''" add sketch "Sketch1 (5)" along normal blind 4 from surface at 1.5 separate body contours L4 L5 L6 L7 | A0 | L10 L11 L14 L15 | A1 | L16 L17 L20 L21 | A2 makes body 75 at (-1, 1, 1.5) makes body 76 at (-16, 1, 1.5) makes body 77 at (14, 1, 1.5) in component "Buttons"
extrude "Extrude3''''" add sketch "Sketch1 (5)" along normal blind 2 from surface at 5.5 contours A0 | A1 | A2 bodies 76 75 77 in component "Buttons"
extrude "Extrude4'''" add sketch "Sketch1 (5)" against normal blind 15 separate body contours L0 L2 L22 L23 L24 L25 makes body 78 in component "Buttons"
sketch "Sketch8" plane through (0, 0, 33) normal (0, 0, -1) x (1, 0, 0) in component "Box"
  line L0 (33, 0.5) -> (-33, 0.5)
  line L1 (-33, 0.5) -> (-33, -71.5)
  line L2 (-33, -71.5) -> (33, -71.5)
  line L3 (33, -71.5) -> (33, 0.5)
  line L4 (-23, -46.5) -> (-23, -61.5)
  line L5 (-23, -61.5) -> (25.5, -61.5)
  line L6 (25.5, -61.5) -> (25.5, -46.5)
  line L7 (25.5, -46.5) -> (-23, -46.5)
  line L8 (-20, -50.5) -> (-23, -50.5)
  line L9 (-23, -50.5) -> (-23, -61.5)
  line L10 (-23, -61.5) -> (-20, -61.5)
  line L11 (-20, -61.5) -> (-20, -50.5)
  line L12 (-18, -56.5) -> (-18, -50.5)
  line L13 (18, -50.5) -> (18, -56.5)
  line L14 (25.5, -46.5) -> (25.5, -61.5)
  line L15 (-12, -50.5) -> (-12, -56.5)
  line L16 (-3, -56.5) -> (-3, -50.5)
  line L17 (3, -50.5) -> (3, -56.5)
  line L18 (12, -56.5) -> (12, -50.5)
  line L19 (-25.5, -64) -> (28, -64)
  line L20 (28, -64) -> (28, -44)
  line L21 (28, -44) -> (-25.5, -44)
  line L22 (-25.5, -44) -> (-25.5, -64)
  line L23 (-23.5, -62) -> (26, -62)
  line L24 (26, -62) -> (26, -46)
  line L25 (26, -46) -> (-23.5, -46)
  line L26 (-23.5, -46) -> (-23.5, -62)
  line L27 (-23.5, -62) -> (-19.5, -62)
  line L28 (-19.5, -62) -> (-19.5, -50)
  line L29 (-19.5, -50) -> (-23.5, -50)
  line L30 (-23.5, -50) -> (-23.5, -62)
  line L31 (-20, -50.5) -> (-23, -50.5)
  line L32 (-20, -61.5) -> (-20, -50.5)
  circle A0 centre (15, -53.5) radius 1.5 construction
  circle A1 centre (0, -53.5) radius 1.5 construction
  circle A2 centre (-15, -53.5) radius 1.5 construction
  line L33 (-15, -53.5) -> (15, -53.5) construction
  line L34 (-35, -73.5) -> (35, -73.5) construction
  dimension "d213" = 2.5
  dimension "d214" = 0.5
  dimension "d217" = 0.5
  dimension "d218" = 0.5
  dimension "d254" = 20
  constraint horizontal L27
  constraint vertical L28
  constraint horizontal L29
  constraint vertical L30
  constraint coincident A2.centre L33.start
  constraint coincident A0.centre L33.end
  measures "d217" distance of L29 L31
  measures "d218" distance of L28 L32
  measures "d254" distance of L33 L34
extrude "Extrude10" add sketch "Sketch8" along normal up to surface (4.5 mm away) contours L19 L20 L21 L22 bodies 67 in component "Box"
extrude "Extrude11" add sketch "Sketch8" along normal blind 2 from surface at 4.5 contours L4 L5 L6 L7 L14 L23 L24 L25 L26 L28 L29 | L4 L5 L6 L7 L14 L28 L29 | L19 L20 L21 L22 bodies 67 in component "Box"
sketch "Sketch7" plane through (0, 0, 35) normal (0, 0, 1) x (-1, 0, 0) in component "Box"
  line L0 (35, -71.5) -> (35, 2.5)
  line L1 (35, 2.5) -> (-35, 2.5)
  line L2 (-35, 2.5) -> (-35, -71.5)
  line L3 (-35, -71.5) -> (35, -71.5)
  line L4 (25.5, -64) -> (-28, -64)
  line L5 (25.5, -44) -> (25.5, -64)
  line L6 (-28, -44) -> (25.5, -44)
  line L7 (-28, -64) -> (-28, -44)
  line L8 (-26, -62) -> (-26, -46)
  line L9 (-26, -46) -> (23.5, -46)
  line L10 (23.5, -62) -> (-26, -62)
  line L11 (23.5, -46) -> (23.5, -62)
  line L12 (24.5, -63) -> (-27, -63)
  line L13 (24.5, -45) -> (24.5, -63)
  line L14 (-27, -45) -> (24.5, -45)
  line L15 (-27, -63) -> (-27, -45)
  dimension "d226" = 1
  dimension "d227" = 1
  dimension "d229" = 1
  dimension "d230" = 1
  constraint parallel L11 L13
  constraint parallel L10 L12
  constraint parallel L9 L14
  constraint parallel L8 L15
  measures "d226" distance of L10 L12
  measures "d227" distance of L11 L13
  measures "d229" distance of L8 L15
  measures "d230" distance of L9 L14
extrude "Extrude12" cut sketch "Sketch7" against normal blind 1 contours L8 L9 L10 L11 | L12 L13 L14 L15 bodies 67 in component "Box"
extrude "Extrude13" cut sketch "Sketch7" against normal blind 2 contours L8 L9 L10 L11 bodies 67 in component "Box"
sketch "Sketch9" plane through (0, 0, 28.5) normal (0, 0, 1) x (-1, 0, 0) in component "Box"
  line L0 (-26, -62) -> (19.5, -62)
  line L1 (19.5, -62) -> (19.5, -50)
  line L2 (19.5, -50) -> (23.5, -50)
  line L3 (23.5, -50) -> (23.5, -46)
  line L4 (23.5, -46) -> (-26, -46)
  line L5 (-26, -46) -> (-26, -62)
  line L6 (12, -50.5) -> (12, -56.5)
  line L7 (3, -56.5) -> (3, -50.5)
  line L8 (-3, -50.5) -> (-3, -56.5)
  line L9 (-12, -56.5) -> (-12, -50.5)
  line L10 (-18, -50.5) -> (-18, -56.5)
  line L11 (23, -61.5) -> (23, -46.5)
  line L12 (23, -46.5) -> (-25.5, -46.5)
  line L13 (-25.5, -46.5) -> (-25.5, -61.5)
  line L14 (-25.5, -61.5) -> (23, -61.5)
  line L15 (20, -61.5) -> (20, -50.5)
  line L16 (13, -46) -> (13, -62)
  line L17 (17, -62) -> (17, -46)
  line L18 (-2, -46) -> (-2, -62)
  line L19 (2, -62) -> (2, -46)
  line L20 (-22, -62) -> (-22, -46)
  line L21 (-17, -62) -> (-17, -46)
  line L22 (-13, -46) -> (-13, -62)
  line L23 (23.5, -62) -> (-26, -62)
  line L24 (-26, -46) -> (23.5, -46)
  line L25 (-26, -62) -> (-26, -46)
  dimension "d236" = 1
  dimension "d237" = 1
  dimension "d238" = 1
  dimension "d242" = 4
  dimension "d243" = 1
  dimension "d244" = 1
  dimension "d245" = 4
  constraint vertical L16
  constraint vertical L17
  constraint vertical L18
  constraint vertical L19
  constraint vertical L20
  constraint vertical L21
  constraint vertical L22
  constraint coincident L0 L17.start
  constraint coincident L0 L16.end
  constraint coincident L0 L19.start
  constraint coincident L0 L18.end
  constraint coincident L0 L22.end
  constraint coincident L0 L21.start
  constraint coincident L0 L20.start
  constraint coincident L4 L20.end
  constraint coincident L4 L21.end
  constraint coincident L4 L22.start
  constraint coincident L4 L18.start
  constraint coincident L4 L19.end
  constraint coincident L4 L16.start
  constraint coincident L4 L17.end
  measures "d236" distance of L6 L16
  measures "d237" distance of L7 L19
  measures "d238" distance of L8 L18
  measures "d242" distance of L16 L17
  measures "d243" distance of L9 L22
  measures "d244" distance of L10 L21
  measures "d245" distance of L20 L25
extrude "Extrude14" add sketch "Sketch9" along normal up to surface (0.75 mm away) contours L0 L4 L5 L12 L13 L14 L20 L23 L24 L25 | L0 L14 L21 L22 L23 | L12 L13 L14 L20 | L12 L14 L21 L22 | L4 L12 L21 L22 L24 | L0 L14 L18 L19 L23 | L12 L14 L18 L19 | L4 L12 L18 L19 L24 | L0 L14 L16 L17 L23 | L12 L14 L16 L17 | L4 L12 L16 L17 L24 bodies 67 in component "Box"
fillet "Fillet1" radius 1 4 edges at (-19.3, 6.8, -33) (8.6, 6.8, -33) (-21.9692, 56.296, -33) (26.6308, 55.096, -33) on bodies 67 in component "Box"
fillet "Fillet1" radius 1 12 edges at (1.25, 64, 33) (28, 54, 33) (-25.5, 54, 33) (1.25, 44, 33) (-25.5, 64, 29.75) (-25.5, 44, 29.75) (-25.5, 54, 26.5) (1.25, 64, 26.5) (28, 64, 29.75) (28, 54, 26.5) (28, 44, 29.75) (1.25, 44, 26.5) on bodies 67 in component "Box"
sketch "Sketch1 (6)" plane through (0, 0, 35) normal (0, 0, 1) x (-1, 0, 0) in component "Cap"
  line L0 (24.5, -45) -> (24.5, -63) construction
  line L1 (24.5, -63) -> (-27, -63) construction
  line L2 (-27, -63) -> (-27, -45) construction
  line L3 (-27, -45) -> (24.5, -45) construction
  line L4 (35, -71.5) -> (35, 2.5)
  line L5 (35, 2.5) -> (-35, 2.5)
  line L6 (-35, 2.5) -> (-35, -71.5)
  line L7 (-35, -71.5) -> (35, -71.5)
  line L8 (-26, -62) -> (-26, -46) construction
  line L9 (-26, -46) -> (23.5, -46) construction
  line L10 (23.5, -46) -> (23.5, -62) construction
  line L11 (23.5, -62) -> (-26, -62) construction
  line L12 (-27, -63) -> (24.5, -63) construction
  line L13 (24.5, -63) -> (24.5, -45) construction
  line L14 (24.5, -45) -> (-27, -45) construction
  line L15 (-27, -45) -> (-27, -63) construction
  circle A0 centre (-15, -53.5) radius 1.5 construction
  circle A1 centre (-15, -53.5) radius 1.5 construction
  line L16 (-12, -50.5) -> (-18, -50.5) construction
  line L17 (-18, -50.5) -> (-18, -56.5) construction
  line L18 (-18, -56.5) -> (-12, -56.5) construction
  line L19 (-12, -56.5) -> (-12, -50.5) construction
  circle A2 centre (0, -53.5) radius 1.5 construction
  line L20 (3, -50.5) -> (-3, -50.5) construction
  line L21 (-3, -50.5) -> (-3, -56.5) construction
  line L22 (-3, -56.5) -> (3, -56.5) construction
  line L23 (3, -56.5) -> (3, -50.5) construction
  circle A3 centre (15, -53.5) radius 1.5 construction
  line L24 (18, -50.5) -> (12, -50.5) construction
  line L25 (12, -50.5) -> (12, -56.5) construction
  line L26 (12, -56.5) -> (18, -56.5) construction
  line L27 (18, -56.5) -> (18, -50.5) construction
  line L28 (24.25, -45.25) -> (-26.75, -45.25)
  line L29 (-26.75, -45.25) -> (-26.75, -62.75)
  line L30 (-26.75, -62.75) -> (24.25, -62.75)
  line L31 (24.25, -62.75) -> (24.25, -45.25)
  line L32 (18.25, -50.25) -> (11.75, -50.25)
  line L33 (11.75, -50.25) -> (11.75, -56.75)
  line L34 (11.75, -56.75) -> (18.25, -56.75)
  line L35 (18.25, -56.75) -> (18.25, -50.25)
  line L36 (3.25, -50.25) -> (-3.25, -50.25)
  line L37 (-3.25, -50.25) -> (-3.25, -56.75)
  line L38 (-3.25, -56.75) -> (3.25, -56.75)
  line L39 (3.25, -56.75) -> (3.25, -50.25)
  line L40 (-11.75, -50.25) -> (-18.25, -50.25)
  line L41 (-18.25, -50.25) -> (-18.25, -56.75)
  line L42 (-18.25, -56.75) -> (-11.75, -56.75)
  line L43 (-11.75, -56.75) -> (-11.75, -50.25)
  line L44 (-25.75, -46.25) -> (23.25, -46.25)
  line L45 (23.25, -46.25) -> (23.25, -61.75)
  line L46 (23.25, -61.75) -> (-25.75, -61.75)
  line L47 (-25.75, -61.75) -> (-25.75, -46.25)
  dimension "d260" = -0.25
  dimension "d261" = 0.25
  dimension "d262" = 0.25
  dimension "d263" = 0.25
  dimension "d264" = 0.25
extrude "Extrude1'''''" add sketch "Sketch1 (6)" against normal up to surface (0.75 mm away) separate body contours L28 L29 L30 L31 | L44 L45 L46 L47 makes body 79 in component "Cap"
extrude "Extrude2'''''" add sketch "Sketch1 (6)" against normal blind 2 from surface at -0.75 contours L44 L45 L46 L47 bodies 79 in component "Cap"
draft "Draft1'" angle 11.25 neutral plane through (0, 0, 34.25) pull (0, 0, -1) 4 faces at (9.4167, 46.25, 33.5833) (-23.25, 51.4167, 33.5833) (-6.9167, 61.75, 33.5833) (25.75, 56.5833, 33.5833) on bodies 79 in component "Cap"
component "LED Matrix" placed x (1, 0, 0) y (0, 1, 0) z (0, 0, 1) at (0, 0, 0)
component "Box" placed x (1, 0, 0) y (0, 1, 0) z (0, 0, 1) at (0, 0, 0)
component "Arduino" placed x (1, 0, 0) y (0, 1, 0) z (0, 0, 1) at (0, 36.5, 5)
component "Door" placed x (1, 0, 0) y (0, 1, 0) z (0, 0, 1) at (0, 0, 0)
component "Buttons" placed x (1, 0, 0) y (0, 1, 0) z (0, 0, 1) at (0, 53.5, 29.5)
component "Cap" placed x (1, 0, 0) y (0, 1, 0) z (0, 0, 1) at (0, 0, 0)
equation "d54 = d50"
equation "d57 = d50"
equation "d171 = d170"
equation "d172 = d170"
equation "d173 = d170"
equation "d262 = d261"
equation "d263 = d261"
named bodies: "Box", "Door", "Cap"
